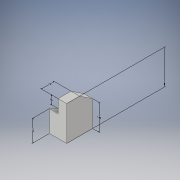
# Autodesk Inventor part: AW7.14
Saved by Autodesk Inventor 2018 (Build 220112000, 112)
## iProperties
Created: 2019-01-22
Part Number: AW7.14
Material: Generic
Document SubType Name: Modeling
Designer: russd
Density: 1 g/cm^3
Appearance: Default
Author: russd
Autodesk Inventor part; units mm, degrees
ref_plane "YZ Plane" through (0, 0, 0) normal (1, 0, 0) x (0, 1, 0)
ref_plane "XZ Plane" through (0, 0, 0) normal (0, 1, 0) x (-1, 0, 0)
ref_plane "XY Plane" through (0, 0, 0) normal (0, 0, 1) x (1, 0, 0)
sketch "Sketch1" plane through (0, 0, 0) normal (0, 0, 1) x (1, 0, 0)
  point P0 (0, 0)
sketch "Sketch2" plane through (0, 0, 0) normal (0, 0, 1) x (1, 0, 0)
  line L0 (-1.5778, 19.1305) -> (11.1222, 19.1305)
  line L1 (11.1222, 19.1305) -> (11.1222, -31.6695)
  line L2 (11.1222, -31.6695) -> (-1.5778, -31.6695)
  line L3 (-1.5778, 0.0805) -> (-1.5778, 19.1305)
  line L4 (11.1222, -31.6695) -> (-14.2778, -31.6695)
  line L5 (-14.2778, -31.6695) -> (-14.2778, 0.0805)
  line L6 (-14.2778, 0.0805) -> (-1.5778, 0.0805)
  line L7 (11.1222, 0.0805) -> (11.1222, -31.6695)
  line L8 (-1.5778, 0.0805) -> (-1.5778, -31.6695)
  point P0 (0, 0)
  dimension "d0" = 12.7
  dimension "d1" = 50.8
  dimension "d2" = 25.4
  dimension "d3" = 31.75
  constraints: 18 end point, 4 parallel, 3 perpendicular, 2 horizontal
  measures "d0" distance of L1.end L2.end
  measures "d1" distance of L0.end L1.end
  measures "d2" distance of L5.end L7.start
  measures "d3" distance of L4.end L5.end
extrude "Extrusion1" add sketch "Sketch2" along normal blind 38.1
draft "FaceDraft2" angle 26.5 pull direction (0, 0, -1) fixed plane through (-1.5778, -21.0862, 38.1) normal (0, 0, 1) faces at (-10.0445, 0.0805, 12.7)
chamfer "Chamfer1" distance 19.05 angle 33.6 1 edges at (4.7722, 19.1305, 0) measured on face at (4.7722, 19.1305, 0.5)
body "Solid1"
